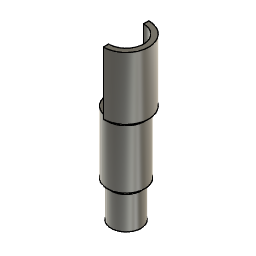
Photoreactor Probe v2 (Autodesk Fusion 360 design; units mm, degrees)
Autodesk Fusion 360 part; units mm, degrees
sketch "Sketch1" plane through (0, 0, 0) normal (0, 0, 1) x (1, 0, 0)
  circle A0 centre (0, 0) radius 5.75
  circle A1 centre (0, 0) radius 3.75
  dimension "d1" = 11.5
  dimension "d2" = 7.5
  constraint coincident A0.centre A1.centre
  constraint concentric A0 A1
  measures "d1" diameter of A0
  measures "d2" diameter of A1
extrude "Extrude1" add sketch "Sketch1" along normal blind 20
sketch "Sketch2" plane through (0, 0, 20) normal (0, 0, 1) x (-1, 0, 0)
  circle A0 centre (0, 0) radius 3.75
  circle A1 centre (0, 0) radius 5.75
  circle A2 centre (0, 0) radius 3.75
  circle A3 centre (0, 0) radius 5.25
  circle A4 centre (0, 0) radius 7.25
  dimension "d5" = 10.5
  dimension "d6" = 14.5
  constraint concentric A0 A2
  constraint concentric A0 A3
  constraint concentric A3 A4
  measures "d5" diameter of A3
  measures "d6" diameter of A4
extrude "Extrude2" add sketch "Sketch2" along normal blind 24 contours A1 | A4
sketch "Sketch3" plane through (0, 0, 44) normal (0, 0, 1) x (-1, 0, 0)
  circle A0 centre (0, 0) radius 5.25
  circle A1 centre (0, 0) radius 7.25
  circle A2 centre (0, 0) radius 6.75
  circle A3 centre (0, 0) radius 8.75
  line L0 (0, 5.25) -> (0, 8.75)
  line L1 (0, -5.25) -> (0, -8.75)
  dimension "d9" = 13.5
  dimension "d10" = 17.5
  constraint coincident A0.centre A1.centre
  constraint coincident A0 L0.start
  constraint coincident A3 L0.end
  constraint vertical L0
  constraint coincident A0 L1.start
  constraint coincident A3 L1.end
  constraint vertical L1
  measures "d9" diameter of A2
  measures "d10" diameter of A3
extrude "Extrude3" add sketch "Sketch3" along normal blind 24 contours A1 A2 L0 L1 | A1 A3 L0 L1 picked at (-0.3602, -7.0563) picked at (-0.7949, 8.1904)
chamfer "Chamfer1" distance 1.5 angle 45 1 edges at (7.25, 0, 44)
chamfer "Chamfer2" distance 1.5 angle 45 1 edges at (-5.3609, -2.0793, 20)
extrude "Extrude4" cut 1 faces at (5.048, -0.472, 0) along direction (0, 0, 1) blind 6
